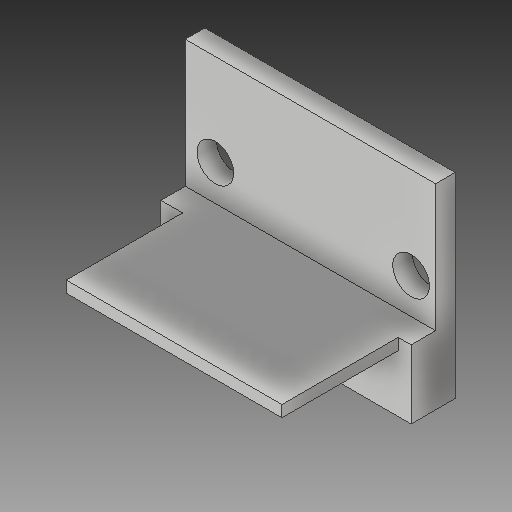
# Autodesk Inventor part: SensorCJMCU530
Saved by Autodesk Inventor 2017 (Build 210142000, 142)
## iProperties
Part Number: SensorCJMCU530
Material: Genérico
Document SubType Name: Modeling
Designer: Leonardo
Density: 1 g/cm^3
Appearance: Valor por defecto
Mass: 0.897727 g
Surface Area: 12.4366 cm^2
Volume: 0.897727 cm^3
Author: Leonardo
Autodesk Inventor part; units mm, degrees
ref_plane "YZ Plane" through (0, 0, 0) normal (1, 0, 0) x (0, 1, 0)
ref_plane "XZ Plane" through (0, 0, 0) normal (0, 1, 0) x (-1, 0, 0)
ref_plane "XY Plane" through (0, 0, 0) normal (0, 0, 1) x (1, 0, 0)
sketch "Boceto1" plane through (0, 0, 0) normal (0, 0, 1) x (1, 0, 0)
  circle A0 centre (20.3885, 0.1002) radius 16.5 projected
  circle A1 centre (20.3885, 0.1002) radius 19.85 projected
  line L0 (10.1635, 8.1002) -> (30.6135, 8.1002)
  line L1 (30.6135, 8.1002) -> (30.6135, -7.8998)
  line L2 (30.6135, -7.8998) -> (10.1635, -7.8998)
  line L3 (10.1635, -7.8998) -> (10.1635, 8.1002)
  line L4 (10.1635, 8.1002) -> (30.6135, -7.8998) construction
  line L5 (30.6135, 8.1002) -> (10.1635, -7.8998) construction
  point P0 (0, 0)
  dimension "d0" = 20.45
  dimension "d1" = 16
  constraints: 12 end point, 2 midpoint, 2 parallel, 1 horizontal, 1 perpendicular
  measures "d0" distance of L1.end L2.end
  measures "d1" distance of L0.end L1.end
extrude "Extrusión1" add sketch "Boceto1" along normal blind 1.6 contours L0 L1 L2 L3
sketch "Boceto2" plane through (0, 0, 1.6) normal (0, 0, 1) x (1, 0, 0)
  line L0 (10.1635, -7.8998) -> (30.6135, -7.8998) projected
  line L1 (30.6135, -7.8998) -> (30.6135, -2.2998)
  line L2 (30.6135, -7.8998) -> (30.6135, 8.1002) projected
  line L3 (30.6135, -2.2998) -> (10.1635, -2.2998)
  line L4 (10.1635, 8.1002) -> (10.1635, -7.8998) projected
  line L5 (10.1635, -7.8998) -> (10.1635, -2.2998)
  line L6 (30.6135, -7.8998) -> (10.1635, -7.8998)
  point P0 (0, 0)
  dimension "d4" = 5.6
  constraints: 8 end point, 2 perpendicular, 2 point on line, 1 collinear
  measures "d4" distance of L0.end L1.end
extrude "Extrusión2" add sketch "Boceto2" along normal blind 11.5
sketch "Boceto3" plane through (0, 0, 13.1) normal (0, 0, 1) x (1, 0, 0)
  line L0 (30.6135, -2.2998) -> (10.1635, -2.2998) projected
  line L1 (11.9387, -2.2998) -> (10.1635, -2.2998)
  line L2 (10.1635, -2.2998) -> (10.1635, -7.8194)
  line L3 (10.1635, -7.8194) -> (30.6135, -7.8194)
  line L4 (30.6135, -7.8194) -> (30.6135, -2.2998)
  line L5 (30.6135, -2.2998) -> (29.5577, -2.2998)
  line L6 (29.5577, -3.2351) -> (11.9387, -3.2351)
  line L7 (11.9387, -3.2351) -> (11.9387, -2.2998)
  line L8 (29.5577, -2.2998) -> (29.5577, -3.2351)
  point P0 (0, 0)
  constraints: 16 end point, 4 perpendicular, 2 point on line, 1 collinear, 1 horizontal, 1 parallel
extrude "Extrusión3" cut sketch "Boceto3" against normal blind 9.5 contours L4 L3 L2 L0 L7 L6 L8
sketch "Boceto4" plane through (0, 0, 13.1) normal (0, 0, 1) x (1, 0, 0)
  line L0 (30.6135, -7.8194) -> (10.1635, -7.8194) projected
  line L1 (10.1635, -7.8194) -> (10.1635, -7.8998) projected
  line L2 (10.1635, -7.8998) -> (30.6135, -7.8998) projected
  line L3 (30.6135, -7.8998) -> (30.6135, -7.8194) projected
  point P0 (0, 0)
extrude "Extrusión4" cut sketch "Boceto4" against normal blind 9.5
sketch "Boceto5" plane through (0, 0, 1.6) normal (0, 0, 1) x (1, 0, 0)
  circle A0 centre (28.6135, 0.6002) radius 1.5
  line L0 (28.6135, 0.6002) -> (12.6135, 0.6002) construction
  line L1 (28.6135, 0.6002) -> (44.6135, 0.6002) construction
  circle A1 centre (12.6135, 0.6002) radius 1.5
  point P0 (0, 0)
  point P1 (30.6135, 8.1002)
  dimension "d14" = 16
  dimension "d15" = 180
  dimension "d16" = 3
  constraints: 4 end point, 2 centre point, 2 horizontal, 1 coincident, 1 collinear
  measures "d14" distance of L0.start L0.end
  measures "d15" angle of L0 L1
  measures "d16" diameter of A1
extrude "Extrusión5" cut sketch "Boceto5" against normal through all
sketch "Boceto6" plane through (0, 0, 0) normal (0, 0, -1) x (-1, 0, 0)
  line L0 (-10.1635, -7.8998) -> (-10.1635, 8.1002) construction
  line L1 (-30.6135, -7.8998) -> (-10.1635, -7.8998) construction
  line L2 (-10.1635, 8.1002) -> (-30.6135, -7.8998) construction
  line L3 (-30.6135, 8.1002) -> (-30.6135, -7.8998) construction
  line L4 (-10.1635, -7.8998) -> (-30.6135, 8.1002) construction
  line L5 (-19.1385, 2.3502) -> (-21.6385, 2.3502)
  line L6 (-21.6385, 2.3502) -> (-21.6385, -2.1498)
  line L7 (-21.6385, -2.1498) -> (-19.1385, -2.1498)
  line L8 (-19.1385, -2.1498) -> (-19.1385, 2.3502)
  line L9 (-19.1385, 2.3502) -> (-21.6385, -2.1498) construction
  line L10 (-21.6385, 2.3502) -> (-19.1385, -2.1498) construction
  point P0 (0, 0)
  point P1 (-20.3885, 0.1002)
  dimension "d19" = 2.5
  dimension "d20" = 4.5
  constraints: 16 end point, 3 midpoint, 2 parallel, 1 horizontal, 1 perpendicular
  measures "d19" distance of L7.end L6.end
  measures "d20" distance of L6.end L5.end
extrude "Extrusión6" add sketch "Boceto6" along normal blind 1
